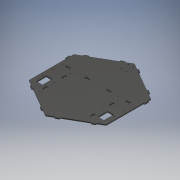
# Autodesk Inventor part: BA20
Saved by Autodesk Inventor 2017 (Build 210142000, 142)
## iProperties
Created: 2019-06-03
Part Number: BA20
Material: Polyethylene, High Density
Document SubType Name: Modeling
Designer: Dell
Density: 0.952 g/cm^3
Appearance: Smooth - Black
Mass: 1382.1 g
Surface Area: 4727.34 cm^2
Volume: 1451.78 cm^3
Author: Dell
Autodesk Inventor part; units mm, degrees
ref_plane "YZ Plane" through (0, 0, 0) normal (1, 0, 0) x (0, 1, 0)
ref_plane "XZ Plane" through (0, 0, 0) normal (0, 1, 0) x (-1, 0, 0)
ref_plane "XY Plane" through (0, 0, 0) normal (0, 0, 1) x (1, 0, 0)
sketch "Sketch1" plane through (0, 0, 0) normal (0, 0, 1) x (1, 0, 0)
  line L0 (0, 303.5592) -> (262.89, 151.7796) construction
  line L1 (262.89, 151.7796) -> (262.89, -151.7796) construction
  line L2 (262.89, -151.7796) -> (0, -303.5592) construction
  line L3 (0, -303.5592) -> (-262.89, -151.7796) construction
  line L4 (-262.89, -151.7796) -> (-262.89, 151.7796) construction
  line L5 (-262.89, 151.7796) -> (0, 303.5592) construction
  line L6 (0, 296.2269) -> (256.54, 148.1134)
  line L7 (256.54, 148.1134) -> (256.54, -148.1134)
  line L8 (256.54, -148.1134) -> (0, -296.2269)
  line L9 (0, -296.2269) -> (-256.54, -148.1134)
  line L10 (-256.54, -148.1134) -> (-256.54, 148.1134)
  line L11 (-256.54, 148.1134) -> (0, 296.2269)
  point P0 (0, 0)
  point P1 (0, 0)
  point P2 (262.89, 0)
  dimension "d0" = 525.78
  dimension "d1" = 6.35
  constraints: 24 end point, 1 coincident, 1 horizontal alignment, 1 midpoint, 18 other
  measures "d0" distance between parallel lines of L1 L4
  measures "d1" distance between parallel lines of L4 L10
extrude "Extrusion1" add sketch "Sketch1" along normal blind 6.35
sketch "Sketch2" plane through (0, 0, 6.35) normal (0, 0, 1) x (1, 0, 0)
  line L0 (-212.09, 56.5296) -> (-186.69, 56.5296)
  line L1 (-186.69, 56.5296) -> (-186.69, 50.1796)
  line L2 (-186.69, 50.1796) -> (-212.09, 50.1796)
  line L3 (-212.09, 50.1796) -> (-212.09, 56.5296)
  line L4 (256.54, 148.1134) -> (0, 296.2269) construction
  line L5 (0, 296.2269) -> (-256.54, 148.1134) construction
  line L6 (-256.54, 148.1134) -> (-256.54, -148.1134) construction
  line L7 (-256.54, -148.1134) -> (0, -296.2269) construction
  line L8 (0, -296.2269) -> (256.54, -148.1134) construction
  line L9 (256.54, -148.1134) -> (256.54, 148.1134) construction
  line L10 (-262.89, 151.7796) -> (0, 303.5592) construction
  line L11 (0, 303.5592) -> (262.89, 151.7796) construction
  line L12 (262.89, 151.7796) -> (262.89, -151.7796) construction
  line L13 (262.89, -151.7796) -> (0, -303.5592) construction
  line L14 (0, -303.5592) -> (-262.89, -151.7796) construction
  line L15 (-262.89, -151.7796) -> (-262.89, 151.7796) construction
  line L16 (-85.09, 50.1796) -> (-59.69, 50.1796)
  line L17 (-59.69, 50.1796) -> (-59.69, 56.5296)
  line L18 (-59.69, 56.5296) -> (-85.09, 56.5296)
  line L19 (-85.09, 56.5296) -> (-85.09, 50.1796)
  line L20 (0, 0) -> (0, 303.5592) construction
  line L21 (212.09, 56.5296) -> (186.69, 56.5296)
  line L22 (186.69, 56.5296) -> (186.69, 50.1796)
  line L23 (186.69, 50.1796) -> (212.09, 50.1796)
  line L24 (212.09, 50.1796) -> (212.09, 56.5296)
  line L25 (85.09, 50.1796) -> (59.69, 50.1796)
  line L26 (59.69, 50.1796) -> (59.69, 56.5296)
  line L27 (59.69, 56.5296) -> (85.09, 56.5296)
  line L28 (85.09, 56.5296) -> (85.09, 50.1796)
  point P0 (-186.69, 53.3546)
  point P1 (-85.09, 53.3546)
  point P2 (186.69, 53.3546)
  point P3 (85.09, 53.3546)
  dimension "d4" = 6.35
  dimension "d6" = 50.8
  dimension "d7" = 6.35
  dimension "d8" = 25.4
  dimension "d9" = 25.4
  dimension "d10" = 101.6
  dimension "d13" = 101.6
  constraints: 46 end point, 10 symmetric about line, 4 parallel, 2 horizontal, 2 horizontal alignment, 2 midpoint, 2 perpendicular, 1 vertical, 5 other
  measures "d4" distance between parallel lines of L5 L10
  measures "d6" distance between parallel lines of L15 L3
  measures "d7" distance of L2.end L0.start
  measures "d8" distance of L0.start L0.end
  measures "d9" distance of L17.end L18.end
  measures "d10" distance between parallel lines of L1 L19
  measures "d13" distance from line of L10.start L2
extrude "Extrusion2" cut sketch "Sketch2" against normal through all
sketch "Sketch3" plane through (0, 0, 6.35) normal (0, 0, 1) x (1, 0, 0)
  line L0 (-161.29, -0.6204) -> (-154.94, -0.6204)
  line L1 (-154.94, -0.6204) -> (-154.94, -26.0204)
  line L2 (-154.94, -26.0204) -> (-161.29, -26.0204)
  line L3 (-161.29, -26.0204) -> (-161.29, -0.6204)
  line L4 (-186.69, 50.1796) -> (-212.09, 50.1796) projected
  line L5 (-161.29, -127.6204) -> (-154.94, -127.6204)
  line L6 (-154.94, -127.6204) -> (-154.94, -153.0204)
  line L7 (-154.94, -153.0204) -> (-161.29, -153.0204)
  line L8 (-161.29, -153.0204) -> (-161.29, -127.6204)
  line L9 (-256.54, 148.1134) -> (-256.54, -148.1134) projected
  line L10 (0, 0) -> (0, 56.7776) construction
  line L11 (161.29, -0.6204) -> (154.94, -0.6204)
  line L12 (154.94, -0.6204) -> (154.94, -26.0204)
  line L13 (154.94, -26.0204) -> (161.29, -26.0204)
  line L14 (161.29, -26.0204) -> (161.29, -0.6204)
  line L15 (161.29, -127.6204) -> (154.94, -127.6204)
  line L16 (154.94, -127.6204) -> (154.94, -153.0204)
  line L17 (154.94, -153.0204) -> (161.29, -153.0204)
  line L18 (161.29, -153.0204) -> (161.29, -127.6204)
  dimension "d14" = 6.35
  dimension "d15" = 25.4
  dimension "d16" = 50.8
  dimension "d17" = 6.35
  dimension "d18" = 25.4
  dimension "d19" = 101.6
  dimension "d20" = 95.25
  constraints: 34 end point, 8 symmetric about line, 4 parallel, 2 horizontal, 2 perpendicular, 1 vertical, 1 vertical alignment
  measures "d14" distance of L1.end L2.end
  measures "d15" distance of L2.end L0.start
  measures "d16" distance between parallel lines of L0 L4
  measures "d17" distance of L6.end L7.end
  measures "d18" distance of L5.end L6.end
  measures "d19" distance of L5.start L2.end
  measures "d20" distance between parallel lines of L9 L3
extrude "Extrusion3" cut sketch "Sketch3" along normal through all both and the other way through all
sketch "Sketch4" plane through (0, 0, 6.35) normal (0, 0, 1) x (1, 0, 0)
  line L0 (-264.16, 126.3796) -> (-256.54, 126.3796)
  line L1 (-256.54, 126.3796) -> (-256.54, 100.9796)
  line L2 (-256.54, 100.9796) -> (-264.16, 100.9796)
  line L3 (-264.16, 100.9796) -> (-264.16, 126.3796)
  line L4 (-220.0682, -177.9693) -> (-216.2582, -171.3702)
  line L5 (-216.2582, -171.3702) -> (-194.2611, -184.0702)
  line L6 (-194.2611, -184.0702) -> (-198.0711, -190.6693)
  line L7 (-198.0711, -190.6693) -> (-220.0682, -177.9693)
  line L8 (-62.2789, -260.2702) -> (-66.0889, -266.8693)
  line L9 (-66.0889, -266.8693) -> (-44.0918, -279.5693)
  line L10 (-44.0918, -279.5693) -> (-40.2818, -272.9702)
  line L11 (-40.2818, -272.9702) -> (-62.2789, -260.2702)
  line L12 (-256.54, 148.1134) -> (-256.54, -148.1134) projected
  line L13 (-256.54, -148.1134) -> (0, -296.2269) projected
  line L14 (-196.1661, -187.3697) -> (-64.1839, -263.5697) construction
  line L15 (-130.175, -225.4697) -> (-128.27, -222.1702)
  line L16 (-212.09, 56.5296) -> (-186.69, 56.5296) projected
  line L17 (-186.69, 50.1796) -> (-212.09, 50.1796) projected
  line L18 (0, 0) -> (-92.269, 0) construction
  line L19 (-220.0682, 177.9693) -> (-216.2582, 171.3702)
  line L20 (-216.2582, 171.3702) -> (-194.2611, 184.0702)
  line L21 (-194.2611, 184.0702) -> (-198.0711, 190.6693)
  line L22 (-198.0711, 190.6693) -> (-220.0682, 177.9693)
  line L23 (-62.2789, 260.2702) -> (-66.0889, 266.8693)
  line L24 (-66.0889, 266.8693) -> (-44.0918, 279.5693)
  line L25 (-44.0918, 279.5693) -> (-40.2818, 272.9702)
  line L26 (-40.2818, 272.9702) -> (-62.2789, 260.2702)
  line L27 (-256.54, 148.1134) -> (0, 296.2269)
  line L28 (-196.1661, 187.3697) -> (-64.1839, 263.5697) construction
  line L29 (-130.175, 225.4697) -> (-128.27, 222.1702)
  line L30 (0, 0) -> (0, -66.9145) construction
  line L31 (264.16, 126.3796) -> (256.54, 126.3796)
  line L32 (256.54, 126.3796) -> (256.54, 100.9796)
  line L33 (256.54, 100.9796) -> (264.16, 100.9796)
  line L34 (264.16, 100.9796) -> (264.16, 126.3796)
  line L35 (220.0682, -177.9693) -> (216.2582, -171.3702)
  line L36 (216.2582, -171.3702) -> (194.2611, -184.0702)
  line L37 (194.2611, -184.0702) -> (198.0711, -190.6693)
  line L38 (198.0711, -190.6693) -> (220.0682, -177.9693)
  line L39 (62.2789, -260.2702) -> (66.0889, -266.8693)
  line L40 (66.0889, -266.8693) -> (44.0918, -279.5693)
  line L41 (44.0918, -279.5693) -> (40.2818, -272.9702)
  line L42 (40.2818, -272.9702) -> (62.2789, -260.2702)
  line L43 (256.54, 148.1134) -> (256.54, -148.1134)
  line L44 (196.1661, -187.3697) -> (64.1839, -263.5697) construction
  line L45 (130.175, -225.4697) -> (128.27, -222.1702)
  line L46 (212.09, 56.5296) -> (186.69, 56.5296)
  line L47 (186.69, 50.1796) -> (212.09, 50.1796)
  line L48 (198.0711, 190.6693) -> (220.0682, 177.9693)
  line L49 (220.0682, 177.9693) -> (216.2582, 171.3702)
  line L50 (216.2582, 171.3702) -> (194.2611, 184.0702)
  line L51 (194.2611, 184.0702) -> (198.0711, 190.6693)
  line L52 (130.175, 225.4697) -> (128.27, 222.1702)
  line L53 (196.1661, 187.3697) -> (64.1839, 263.5697) construction
  line L54 (62.2789, 260.2702) -> (66.0889, 266.8693)
  line L55 (40.2818, 272.9702) -> (62.2789, 260.2702)
  line L56 (66.0889, 266.8693) -> (44.0918, 279.5693)
  line L57 (44.0918, 279.5693) -> (40.2818, 272.9702)
  point P0 (92.269, 0)
  dimension "d23" = 7.62
  dimension "d24" = 25.4
  dimension "d25" = 7.62
  dimension "d26" = 25.4
  dimension "d27" = 25.4
  dimension "d28" = 7.62
  dimension "d29" = 152.4
  dimension "d31" = 50.8
  constraints: 108 end point, 48 symmetric about line, 10 point on line, 6 parallel, 4 midpoint, 4 perpendicular, 2 horizontal, 1 coincident, 1 vertical
  measures "d23" distance of L1.end L2.end
  measures "d24" distance of L0.end L1.end
  measures "d25" distance of L4.start L4.end
  measures "d26" distance of L4.end L5.end
  measures "d27" distance of L8.end L9.end
  measures "d28" distance of L8.start L8.end
  measures "d29" distance of L14.start L14.end
  measures "d31" distance from line of L2.end L17
extrude "Extrusion4" add sketch "Sketch4" against normal blind 6.35
sketch "Sketch5" plane through (0, 0, 6.35) normal (0, 0, 1) x (1, 0, 0)
  line L0 (-15.15, 270.8269) -> (15.15, 270.8269) construction
  line L1 (15.15, 270.8269) -> (15.15, 225.2269) construction
  line L2 (15.15, 225.2269) -> (-15.15, 225.2269) construction
  line L3 (-15.15, 225.2269) -> (-15.15, 270.8269) construction
  circle A0 centre (-15.15, 270.8269) radius 3
  circle A1 centre (15.15, 270.8269) radius 3
  circle A2 centre (15.15, 225.2269) radius 3
  circle A3 centre (-15.15, 225.2269) radius 3
  point P0 (0, 0)
  point P1 (0, 270.8269)
  point P2 (0, 296.2269)
  dimension "d34" = 45.6
  dimension "d35" = 30.3
  dimension "d36" = 25.4
  dimension "d37" = 6
  dimension "d38" = 6
  dimension "d39" = 6
  dimension "d40" = 6
  constraints: 8 end point, 4 centre point, 4 coincident, 2 parallel, 1 horizontal, 1 midpoint, 1 perpendicular, 1 vertical alignment
  measures "d34" distance of L0.end L1.end
  measures "d35" distance of L0.start L0.end
  measures "d36" distance from line of point (0, 296.227) L0
  measures "d37" diameter of A0
  measures "d38" diameter of A1
  measures "d39" diameter of A2
  measures "d40" diameter of A3
extrude "Extrusion5" cut sketch "Sketch5" against normal through all
sketch "Sketch6" plane through (0, 0, 6.35) normal (0, 0, 1) x (1, 0, 0)
  circle A0 centre (-207.1647, -181.0197) radius 2.25
  circle A1 centre (-260.35, 113.6796) radius 2.25
  circle A2 centre (-234.315, 53.3546) radius 2.25
  circle A3 centre (-135.89, 53.3546) radius 2.25
  circle A4 centre (0, 53.3546) radius 2.25
  circle A5 centre (-158.115, -178.9798) radius 2.25
  circle A6 centre (-158.115, -76.8204) radius 2.25
  circle A7 centre (-158.115, 26.3671) radius 2.25
  circle A8 centre (-53.1853, -269.9197) radius 2.25
  circle A9 centre (-207.1647, 181.0197) radius 2.25
  circle A10 centre (-53.1853, 269.9197) radius 2.25
  line L0 (-161.29, -0.6204) -> (-154.94, -0.6204) projected
  line L1 (-59.69, 56.5296) -> (-59.69, 50.1796) projected
  line L2 (-264.16, 126.3796) -> (-264.16, 100.9796) projected
  line L3 (-256.54, 126.3796) -> (-264.16, 126.3796) projected
  line L4 (-212.09, 50.1796) -> (-212.09, 56.5296) projected
  line L5 (-212.09, 53.3546) -> (-256.54, 53.3546)
  line L6 (-256.54, 100.9796) -> (-256.54, -148.1134) projected
  line L7 (-186.69, 56.5296) -> (-186.69, 50.1796) projected
  line L8 (-186.69, 53.3546) -> (-85.09, 53.3546)
  line L9 (-85.09, 50.1796) -> (-85.09, 56.5296) projected
  line L10 (-158.115, -0.6204) -> (-158.115, 53.3546)
  line L11 (-161.29, -26.0204) -> (-154.94, -26.0204) projected
  line L12 (-158.115, -26.0204) -> (-158.115, -127.6204)
  line L13 (-161.29, -127.6204) -> (-154.94, -127.6204) projected
  line L14 (-154.94, -153.0204) -> (-161.29, -153.0204) projected
  line L15 (-158.115, -153.0204) -> (-158.115, -204.9391)
  line L16 (-62.2789, -260.2702) -> (-194.2611, -184.0702) projected
  line L17 (-216.2582, -171.3702) -> (-220.0682, -177.9693) projected
  line L18 (-218.1632, -174.6697) -> (-207.1647, -181.0197) construction
  line L19 (-207.1647, -181.0197) -> (-209.0697, -184.3193) construction
  line L20 (-220.0682, -177.9693) -> (-198.0711, -190.6693) projected
  line L21 (-216.2582, 171.3702) -> (-220.0682, 177.9693) projected
  line L22 (-218.1632, 174.6697) -> (-207.1647, 181.0197) construction
  line L23 (-207.1647, 181.0197) -> (-209.0697, 184.3193) construction
  line L24 (-220.0682, 177.9693) -> (-198.0711, 190.6693) construction
  line L25 (-62.2789, 260.2702) -> (-66.0889, 266.8693) projected
  line L26 (-64.1839, 263.5697) -> (-53.1853, 269.9197) construction
  line L27 (-53.1853, 269.9197) -> (-55.0903, 273.2193) construction
  line L28 (-44.0918, 279.5693) -> (-66.0889, 266.8693) projected
  line L29 (-62.2789, -260.2702) -> (-66.0889, -266.8693) projected
  line L30 (-64.1839, -263.5697) -> (-53.1853, -269.9197) construction
  line L31 (-53.1853, -269.9197) -> (-55.0903, -273.2193) construction
  line L32 (-66.0889, -266.8693) -> (-44.0918, -279.5693) projected
  line L33 (0, 0) -> (0, -97.3082) construction
  circle A11 centre (207.1647, -181.0197) radius 2.25
  circle A12 centre (260.35, 113.6796) radius 2.25
  circle A13 centre (234.315, 53.3546) radius 2.25
  circle A14 centre (135.89, 53.3546) radius 2.25
  circle A15 centre (158.115, -178.9798) radius 2.25
  circle A16 centre (158.115, -76.8204) radius 2.25
  circle A17 centre (158.115, 26.3671) radius 2.25
  circle A18 centre (53.1853, -269.9197) radius 2.25
  circle A19 centre (207.1647, 181.0197) radius 2.25
  circle A20 centre (53.1853, 269.9197) radius 2.25
  line L34 (161.29, -0.6204) -> (154.94, -0.6204)
  line L35 (59.69, 56.5296) -> (59.69, 50.1796)
  line L36 (264.16, 126.3796) -> (264.16, 100.9796)
  line L37 (256.54, 126.3796) -> (264.16, 126.3796)
  line L38 (212.09, 50.1796) -> (212.09, 56.5296)
  line L39 (212.09, 53.3546) -> (256.54, 53.3546)
  line L40 (256.54, 100.9796) -> (256.54, -148.1134)
  line L41 (186.69, 56.5296) -> (186.69, 50.1796)
  line L42 (186.69, 53.3546) -> (85.09, 53.3546)
  line L43 (85.09, 50.1796) -> (85.09, 56.5296)
  line L44 (158.115, -0.6204) -> (158.115, 53.3546)
  line L45 (161.29, -26.0204) -> (154.94, -26.0204)
  line L46 (158.115, -26.0204) -> (158.115, -127.6204)
  line L47 (161.29, -127.6204) -> (154.94, -127.6204)
  line L48 (154.94, -153.0204) -> (161.29, -153.0204)
  line L49 (158.115, -153.0204) -> (158.115, -204.9391)
  line L50 (62.2789, -260.2702) -> (194.2611, -184.0702)
  line L51 (216.2582, -171.3702) -> (220.0682, -177.9693)
  line L52 (218.1632, -174.6697) -> (207.1647, -181.0197) construction
  line L53 (207.1647, -181.0197) -> (209.0697, -184.3193) construction
  line L54 (220.0682, -177.9693) -> (198.0711, -190.6693)
  line L55 (216.2582, 171.3702) -> (220.0682, 177.9693)
  line L56 (218.1632, 174.6697) -> (207.1647, 181.0197) construction
  line L57 (207.1647, 181.0197) -> (209.0697, 184.3193) construction
  line L58 (220.0682, 177.9693) -> (198.0711, 190.6693) construction
  line L59 (62.2789, 260.2702) -> (66.0889, 266.8693)
  line L60 (64.1839, 263.5697) -> (53.1853, 269.9197) construction
  line L61 (53.1853, 269.9197) -> (55.0903, 273.2193) construction
  line L62 (44.0918, 279.5693) -> (66.0889, 266.8693)
  line L63 (62.2789, -260.2702) -> (66.0889, -266.8693)
  line L64 (64.1839, -263.5697) -> (53.1853, -269.9197) construction
  line L65 (53.1853, -269.9197) -> (55.0903, -273.2193) construction
  line L66 (66.0889, -266.8693) -> (44.0918, -279.5693)
  point P0 (-59.69, 53.3546)
  point P1 (-264.16, 113.6796)
  point P2 (-260.35, 126.3796)
  point P3 (-135.89, 53.3546)
  point P4 (-234.315, 53.3546)
  point P5 (59.69, 53.3546)
  point P6 (264.16, 113.6796)
  point P7 (260.35, 126.3796)
  point P8 (158.115, -76.8204)
  point P9 (135.89, 53.3546)
  point P10 (234.315, 53.3546)
  dimension "d43" = 4.5
  dimension "d44" = 4.5
  dimension "d45" = 4.5
  dimension "d46" = 4.5
  dimension "d47" = 4.5
  dimension "d53" = 4.5
  dimension "d54" = 4.5
  dimension "d55" = 4.5
  dimension "d56" = 4.5
  dimension "d57" = 4.5
  dimension "d58" = 4.5
  constraints: 94 end point, 70 symmetric about line, 23 midpoint, 21 centre point, 10 coincident, 9 perpendicular, 8 point on line, 5 vertical alignment, 4 horizontal alignment, 1 horizontal, 1 vertical, 10 other
  measures "d43" diameter of A0
  measures "d44" diameter of A1
  measures "d45" diameter of A2
  measures "d46" diameter of A3
  measures "d47" diameter of A4
  measures "d53" diameter of A5
  measures "d54" diameter of A6
  measures "d55" diameter of A7
  measures "d56" diameter of A8
  measures "d57" diameter of A9
  measures "d58" diameter of A10
extrude "Extrusion6" cut sketch "Sketch6" against normal through all
sketch "Sketch7" plane through (0, 0, 6.35) normal (0, 0, 1) x (1, 0, 0)
  circle A0 centre (-238.84, -7.2826) radius 2.5
  circle A1 centre (-238.84, -74.7826) radius 2.5
  line L0 (-186.69, 50.1796) -> (-212.09, 50.1796) projected
  line L1 (-256.54, 100.9796) -> (-256.54, -148.1134) projected
  line L2 (0, 0) -> (0, 120.453)
  circle A2 centre (238.84, -7.2826) radius 2.5
  circle A3 centre (238.84, -74.7826) radius 2.5
  line L3 (186.69, 50.1796) -> (212.09, 50.1796)
  line L4 (256.54, 100.9796) -> (256.54, -148.1134)
  dimension "d61" = 5
  dimension "d62" = 5
  dimension "d63" = 57.4622
  dimension "d64" = 17.7
  dimension "d65" = 67.5
  constraints: 6 end point, 6 symmetric about line, 4 centre point, 1 vertical, 1 vertical alignment, 2 other
  measures "d61" diameter of A0
  measures "d62" diameter of A1
  measures "d63" distance from line of L0 A0.centre
  measures "d64" distance from line of L1 A0.centre
  measures "d65" distance of A1.centre A0.centre
extrude "Extrusion7" cut sketch "Sketch7" against normal through all
sketch "Sketch8" plane through (0, 0, 6.35) normal (0, 0, 1) x (1, 0, 0)
  circle A0 centre (238.84, -7.2826) radius 2.5 construction
  circle A1 centre (-238.84, -7.2826) radius 2.5 construction
  circle A2 centre (-238.84, -74.7826) radius 2.5 construction
  circle A3 centre (238.84, -74.7826) radius 2.5 construction
  circle A4 centre (207.1647, 181.0197) radius 2.25 construction
  circle A5 centre (207.1647, -181.0197) radius 2.25 construction
  circle A6 centre (158.115, -76.8204) radius 2.25 construction
  circle A7 centre (234.315, 53.3546) radius 2.25 construction
  circle A8 centre (158.115, 26.3671) radius 2.25 construction
  circle A9 centre (-207.1647, 181.0197) radius 2.25 construction
  circle A10 centre (-158.115, 26.3671) radius 2.25 construction
  circle A11 centre (-158.115, -178.9798) radius 2.25 construction
  circle A12 centre (-135.89, 53.3546) radius 2.25 construction
  circle A13 centre (-260.35, 113.6796) radius 2.25 construction
  circle A14 centre (-207.1647, -181.0197) radius 2.25 construction
  circle A15 centre (-234.315, 53.3546) radius 2.25 construction
  circle A16 centre (0, 53.3546) radius 2.25 construction
  circle A17 centre (-158.115, -76.8204) radius 2.25 construction
  circle A18 centre (-53.1853, -269.9197) radius 2.25 construction
  circle A19 centre (-53.1853, 269.9197) radius 2.25 construction
  circle A20 centre (135.89, 53.3546) radius 2.25 construction
  circle A21 centre (260.35, 113.6796) radius 2.25 construction
  circle A22 centre (53.1853, -269.9197) radius 2.25 construction
  circle A23 centre (158.115, -178.9798) radius 2.25 construction
  circle A24 centre (53.1853, 269.9197) radius 2.25 construction
  circle A25 centre (15.15, 225.2269) radius 3 construction
  circle A26 centre (-15.15, 270.8269) radius 3 construction
  circle A27 centre (15.15, 270.8269) radius 3 construction
  circle A28 centre (-15.15, 225.2269) radius 3 construction
  line L0 (161.29, -0.6204) -> (161.29, -26.0204) construction
  line L1 (161.29, -26.0204) -> (154.94, -26.0204) construction
  line L2 (154.94, -26.0204) -> (154.94, -0.6204) construction
  line L3 (154.94, -0.6204) -> (161.29, -0.6204) construction
  line L4 (-154.94, -0.6204) -> (-154.94, -26.0204) construction
  line L5 (-154.94, -26.0204) -> (-161.29, -26.0204) construction
  line L6 (-161.29, -26.0204) -> (-161.29, -0.6204) construction
  line L7 (-161.29, -0.6204) -> (-154.94, -0.6204) construction
  line L8 (-154.94, -127.6204) -> (-154.94, -153.0204) construction
  line L9 (-154.94, -153.0204) -> (-161.29, -153.0204) construction
  line L10 (-161.29, -153.0204) -> (-161.29, -127.6204) construction
  line L11 (-161.29, -127.6204) -> (-154.94, -127.6204) construction
  line L12 (161.29, -127.6204) -> (161.29, -153.0204) construction
  line L13 (161.29, -153.0204) -> (154.94, -153.0204) construction
  line L14 (154.94, -153.0204) -> (154.94, -127.6204) construction
  line L15 (154.94, -127.6204) -> (161.29, -127.6204) construction
  line L16 (85.09, 56.5296) -> (85.09, 50.1796) construction
  line L17 (85.09, 50.1796) -> (59.69, 50.1796) construction
  line L18 (59.69, 50.1796) -> (59.69, 56.5296) construction
  line L19 (59.69, 56.5296) -> (85.09, 56.5296) construction
  line L20 (-212.09, 50.1796) -> (-212.09, 56.5296) construction
  line L21 (-212.09, 56.5296) -> (-186.69, 56.5296) construction
  line L22 (-186.69, 56.5296) -> (-186.69, 50.1796) construction
  line L23 (-186.69, 50.1796) -> (-212.09, 50.1796) construction
  line L24 (-59.69, 56.5296) -> (-59.69, 50.1796) construction
  line L25 (-59.69, 50.1796) -> (-85.09, 50.1796) construction
  line L26 (-85.09, 50.1796) -> (-85.09, 56.5296) construction
  line L27 (-85.09, 56.5296) -> (-59.69, 56.5296) construction
  line L28 (212.09, 50.1796) -> (186.69, 50.1796) construction
  line L29 (186.69, 50.1796) -> (186.69, 56.5296) construction
  line L30 (186.69, 56.5296) -> (212.09, 56.5296) construction
  line L31 (212.09, 56.5296) -> (212.09, 50.1796) construction
  line L32 (256.54, 148.1134) -> (216.2582, 171.3702) construction
  line L33 (216.2582, 171.3702) -> (220.0682, 177.9693) construction
  line L34 (220.0682, 177.9693) -> (198.0711, 190.6693) construction
  line L35 (198.0711, 190.6693) -> (194.2611, 184.0702) construction
  line L36 (194.2611, 184.0702) -> (62.2789, 260.2702) construction
  line L37 (62.2789, 260.2702) -> (66.0889, 266.8693) construction
  line L38 (66.0889, 266.8693) -> (44.0918, 279.5693) construction
  line L39 (44.0918, 279.5693) -> (40.2818, 272.9702) construction
  line L40 (40.2818, 272.9702) -> (0, 296.2269) construction
  line L41 (0, 296.2269) -> (-40.2818, 272.9702) construction
  line L42 (-40.2818, 272.9702) -> (-44.0918, 279.5693) construction
  line L43 (-44.0918, 279.5693) -> (-66.0889, 266.8693) construction
  line L44 (-66.0889, 266.8693) -> (-62.2789, 260.2702) construction
  line L45 (-62.2789, 260.2702) -> (-194.2611, 184.0702) construction
  line L46 (-194.2611, 184.0702) -> (-198.0711, 190.6693) construction
  line L47 (-198.0711, 190.6693) -> (-220.0682, 177.9693) construction
  line L48 (-220.0682, 177.9693) -> (-216.2582, 171.3702) construction
  line L49 (-216.2582, 171.3702) -> (-256.54, 148.1134) construction
  line L50 (-256.54, 148.1134) -> (-256.54, 126.3796) construction
  line L51 (-256.54, 126.3796) -> (-264.16, 126.3796) construction
  line L52 (-264.16, 126.3796) -> (-264.16, 100.9796) construction
  line L53 (-264.16, 100.9796) -> (-256.54, 100.9796) construction
  line L54 (-256.54, 100.9796) -> (-256.54, -148.1134) construction
  line L55 (-256.54, -148.1134) -> (-216.2582, -171.3702) construction
  line L56 (-216.2582, -171.3702) -> (-220.0682, -177.9693) construction
  line L57 (-220.0682, -177.9693) -> (-198.0711, -190.6693) construction
  line L58 (-198.0711, -190.6693) -> (-194.2611, -184.0702) construction
  line L59 (-194.2611, -184.0702) -> (-62.2789, -260.2702) construction
  line L60 (-62.2789, -260.2702) -> (-66.0889, -266.8693) construction
  line L61 (-66.0889, -266.8693) -> (-44.0918, -279.5693) construction
  line L62 (-44.0918, -279.5693) -> (-40.2818, -272.9702) construction
  line L63 (-40.2818, -272.9702) -> (0, -296.2269) construction
  line L64 (0, -296.2269) -> (40.2818, -272.9702) construction
  line L65 (44.0918, -279.5693) -> (40.2818, -272.9702) construction
  line L66 (66.0889, -266.8693) -> (44.0918, -279.5693) construction
  line L67 (62.2789, -260.2702) -> (66.0889, -266.8693) construction
  line L68 (62.2789, -260.2702) -> (194.2611, -184.0702) construction
  line L69 (194.2611, -184.0702) -> (198.0711, -190.6693) construction
  line L70 (198.0711, -190.6693) -> (220.0682, -177.9693) construction
  line L71 (220.0682, -177.9693) -> (216.2582, -171.3702) construction
  line L72 (216.2582, -171.3702) -> (256.54, -148.1134) construction
  line L73 (256.54, -148.1134) -> (256.54, 100.9796) construction
  line L74 (264.16, 100.9796) -> (256.54, 100.9796) construction
  line L75 (264.16, 126.3796) -> (264.16, 100.9796) construction
  line L76 (256.54, 126.3796) -> (264.16, 126.3796) construction
  line L77 (256.54, 126.3796) -> (256.54, 148.1134) construction
  line L78 (-193.4394, 187.137) -> (-65.3457, 261.0919) construction
  line L79 (-65.3457, 261.0919) -> (-69.1557, 267.691) construction
  line L80 (-69.1557, 267.691) -> (-43.2701, 282.6361) construction
  line L81 (-43.2701, 282.6361) -> (-39.4601, 276.037) construction
  line L82 (-39.4601, 276.037) -> (0, 298.8193) construction
  line L83 (0, 298.8193) -> (39.4601, 276.037) construction
  line L84 (39.4601, 276.037) -> (43.2701, 282.6361) construction
  line L85 (43.2701, 282.6361) -> (69.1557, 267.691) construction
  line L86 (69.1557, 267.691) -> (65.3457, 261.0919) construction
  line L87 (65.3457, 261.0919) -> (193.4394, 187.137) construction
  line L88 (193.4394, 187.137) -> (197.2494, 193.7361) construction
  line L89 (197.2494, 193.7361) -> (223.135, 178.791) construction
  line L90 (223.135, 178.791) -> (219.325, 172.1919) construction
  line L91 (219.325, 172.1919) -> (258.7851, 149.4096) construction
  line L92 (258.7851, 149.4096) -> (258.7851, 128.6247) construction
  line L93 (258.7851, 128.6247) -> (266.4051, 128.6247) construction
  line L94 (266.4051, 128.6247) -> (266.4051, 98.7345) construction
  line L95 (266.4051, 98.7345) -> (258.7851, 98.7345) construction
  line L96 (258.7851, 98.7345) -> (258.7851, -149.4096) construction
  line L97 (258.7851, -149.4096) -> (219.325, -172.1919) construction
  line L98 (219.325, -172.1919) -> (223.135, -178.791) construction
  line L99 (223.135, -178.791) -> (197.2494, -193.7361) construction
  line L100 (197.2494, -193.7361) -> (193.4394, -187.137) construction
  line L101 (193.4394, -187.137) -> (65.3457, -261.0919) construction
  line L102 (65.3457, -261.0919) -> (69.1557, -267.691) construction
  line L103 (69.1557, -267.691) -> (43.2701, -282.6361) construction
  line L104 (43.2701, -282.6361) -> (39.4601, -276.037) construction
  line L105 (39.4601, -276.037) -> (0, -298.8193) construction
  line L106 (0, -298.8193) -> (-39.4601, -276.037) construction
  line L107 (-39.4601, -276.037) -> (-43.2701, -282.6361) construction
  line L108 (-43.2701, -282.6361) -> (-69.1557, -267.691) construction
  line L109 (-69.1557, -267.691) -> (-65.3457, -261.0919) construction
  line L110 (-65.3457, -261.0919) -> (-193.4394, -187.137) construction
  line L111 (-193.4394, -187.137) -> (-197.2494, -193.7361) construction
  line L112 (-197.2494, -193.7361) -> (-223.135, -178.791) construction
  line L113 (-223.135, -178.791) -> (-219.325, -172.1919) construction
  line L114 (-219.325, -172.1919) -> (-258.7851, -149.4096) construction
  line L115 (-258.7851, -149.4096) -> (-258.7851, 98.7345) construction
  line L116 (-258.7851, 98.7345) -> (-266.4051, 98.7345) construction
  line L117 (-266.4051, 98.7345) -> (-266.4051, 128.6247) construction
  line L118 (-266.4051, 128.6247) -> (-258.7851, 128.6247) construction
  line L119 (-258.7851, 128.6247) -> (-258.7851, 149.4096) construction
  line L120 (-258.7851, 149.4096) -> (-219.325, 172.1919) construction
  line L121 (-219.325, 172.1919) -> (-223.135, 178.791) construction
  line L122 (-223.135, 178.791) -> (-197.2494, 193.7361) construction
  line L123 (-197.2494, 193.7361) -> (-193.4394, 187.137) construction
  line L124 (-220.0682, -177.9693) -> (-216.2582, -171.3702) projected
  circle A29 centre (-219.325, -172.1919) radius 3.175
  line L125 (-62.2789, -260.2702) -> (-194.2611, -184.0702) projected
  circle A30 centre (-193.4394, -187.137) radius 3.175
  circle A31 centre (-258.7851, 98.7345) radius 3.175
  circle A32 centre (-258.7851, 128.6247) radius 3.175
  circle A33 centre (-219.325, 172.1919) radius 3.175
  circle A34 centre (-193.4394, 187.137) radius 3.175
  circle A35 centre (-65.3457, 261.0919) radius 3.175
  line L126 (0, 296.2269) -> (-40.2818, 272.9702) projected
  circle A36 centre (-39.4601, 276.037) radius 3.175
  circle A37 centre (39.4601, 276.037) radius 3.175
  circle A38 centre (65.3457, 261.0919) radius 3.175
  line L127 (62.2789, 260.2702) -> (194.2611, 184.0702) projected
  circle A39 centre (193.4394, 187.137) radius 3.175
  circle A40 centre (219.325, 172.1919) radius 3.175
  line L128 (256.54, 126.3796) -> (264.16, 126.3796) projected
  circle A41 centre (258.7851, 128.6247) radius 3.175
  circle A42 centre (258.7851, 98.7345) radius 3.175
  circle A43 centre (219.325, -172.1919) radius 3.175
  line L129 (194.2611, -184.0702) -> (198.0711, -190.6693) projected
  circle A44 centre (193.4394, -187.137) radius 3.175
  circle A45 centre (-65.3457, -261.0919) radius 3.175
  line L130 (-44.0918, -279.5693) -> (-40.2818, -272.9702) projected
  circle A46 centre (-39.4601, -276.037) radius 3.175
  circle A47 centre (39.4601, -276.037) radius 3.175
  line L131 (194.2611, -184.0702) -> (62.2789, -260.2702) projected
  circle A48 centre (65.3457, -261.0919) radius 3.175
  line L132 (-213.36, 57.7996) -> (-185.42, 57.7996)
  line L133 (-185.42, 57.7996) -> (-185.42, 48.9096)
  line L134 (-185.42, 48.9096) -> (-213.36, 48.9096)
  line L135 (-213.36, 48.9096) -> (-213.36, 57.7996)
  line L136 (-86.36, 57.7996) -> (-58.42, 57.7996)
  line L137 (-58.42, 57.7996) -> (-58.42, 48.9096)
  line L138 (-58.42, 48.9096) -> (-86.36, 48.9096)
  line L139 (-86.36, 48.9096) -> (-86.36, 57.7996)
  line L140 (58.42, 57.7996) -> (86.36, 57.7996)
  line L141 (86.36, 57.7996) -> (86.36, 48.9096)
  line L142 (86.36, 48.9096) -> (58.42, 48.9096)
  line L143 (58.42, 48.9096) -> (58.42, 57.7996)
  line L144 (185.42, 57.7996) -> (213.36, 57.7996)
  line L145 (213.36, 57.7996) -> (213.36, 48.9096)
  line L146 (213.36, 48.9096) -> (185.42, 48.9096)
  line L147 (185.42, 48.9096) -> (185.42, 57.7996)
  line L148 (153.67, 0.6496) -> (162.56, 0.6496)
  line L149 (162.56, 0.6496) -> (162.56, -27.2904)
  line L150 (162.56, -27.2904) -> (153.67, -27.2904)
  line L151 (153.67, -27.2904) -> (153.67, 0.6496)
  line L152 (153.67, -126.3504) -> (162.56, -126.3504)
  line L153 (162.56, -126.3504) -> (162.56, -154.2904)
  line L154 (162.56, -154.2904) -> (153.67, -154.2904)
  line L155 (153.67, -154.2904) -> (153.67, -126.3504)
  line L156 (-162.56, 0.6496) -> (-153.67, 0.6496)
  line L157 (-153.67, 0.6496) -> (-153.67, -27.2904)
  line L158 (-153.67, -27.2904) -> (-162.56, -27.2904)
  line L159 (-162.56, -27.2904) -> (-162.56, 0.6496)
  line L160 (-162.56, -126.3504) -> (-153.67, -126.3504)
  line L161 (-153.67, -126.3504) -> (-153.67, -154.2904)
  line L162 (-153.67, -154.2904) -> (-162.56, -154.2904)
  line L163 (-162.56, -154.2904) -> (-162.56, -126.3504)
  line L164 (-160.3149, -152.0453) -> (-155.9151, -152.0453)
  line L165 (-155.9151, -152.0453) -> (-155.9151, -128.5955)
  line L166 (-155.9151, -128.5955) -> (-160.3149, -128.5955)
  line L167 (-160.3149, -128.5955) -> (-160.3149, -152.0453)
  line L168 (-160.3149, -25.0453) -> (-155.9151, -25.0453)
  line L169 (-155.9151, -25.0453) -> (-155.9151, -1.5955)
  line L170 (-155.9151, -1.5955) -> (-160.3149, -1.5955)
  line L171 (-160.3149, -1.5955) -> (-160.3149, -25.0453)
  line L172 (-211.1149, 51.1547) -> (-187.6651, 51.1547)
  line L173 (-187.6651, 51.1547) -> (-187.6651, 55.5545)
  line L174 (-187.6651, 55.5545) -> (-211.1149, 55.5545)
  line L175 (-211.1149, 55.5545) -> (-211.1149, 51.1547)
  line L176 (-84.1149, 51.1547) -> (-60.6651, 51.1547)
  line L177 (-60.6651, 51.1547) -> (-60.6651, 55.5545)
  line L178 (-60.6651, 55.5545) -> (-84.1149, 55.5545)
  line L179 (-84.1149, 55.5545) -> (-84.1149, 51.1547)
  line L180 (60.6651, 51.1547) -> (84.1149, 51.1547)
  line L181 (84.1149, 51.1547) -> (84.1149, 55.5545)
  line L182 (84.1149, 55.5545) -> (60.6651, 55.5545)
  line L183 (60.6651, 55.5545) -> (60.6651, 51.1547)
  line L184 (187.6651, 51.1547) -> (211.1149, 51.1547)
  line L185 (211.1149, 51.1547) -> (211.1149, 55.5545)
  line L186 (211.1149, 55.5545) -> (187.6651, 55.5545)
  line L187 (187.6651, 55.5545) -> (187.6651, 51.1547)
  line L188 (160.3149, -25.0453) -> (160.3149, -1.5955)
  line L189 (160.3149, -1.5955) -> (155.9151, -1.5955)
  line L190 (155.9151, -1.5955) -> (155.9151, -25.0453)
  line L191 (155.9151, -25.0453) -> (160.3149, -25.0453)
  line L192 (160.3149, -152.0453) -> (160.3149, -128.5955)
  line L193 (160.3149, -128.5955) -> (155.9151, -128.5955)
  line L194 (155.9151, -128.5955) -> (155.9151, -152.0453)
  line L195 (155.9151, -152.0453) -> (160.3149, -152.0453)
  circle A49 centre (-160.3149, -152.0453) radius 3.175
  circle A50 centre (-155.9151, -152.0453) radius 3.175
  circle A51 centre (-155.9151, -128.5955) radius 3.175
  circle A52 centre (-160.3149, -128.5955) radius 3.175
  circle A53 centre (-160.3149, -25.0453) radius 3.175
  circle A54 centre (-160.3149, -1.5955) radius 3.175
  circle A55 centre (-155.9151, -25.0453) radius 3.175
  circle A56 centre (-155.9151, -1.5955) radius 3.175
  circle A57 centre (-211.1149, 51.1547) radius 3.175
  circle A58 centre (-211.1149, 55.5545) radius 3.175
  circle A59 centre (-187.6651, 51.1547) radius 3.175
  circle A60 centre (-187.6651, 55.5545) radius 3.175
  circle A61 centre (-84.1149, 55.5545) radius 3.175
  circle A62 centre (-84.1149, 51.1547) radius 3.175
  circle A63 centre (-60.6651, 55.5545) radius 3.175
  circle A64 centre (-60.6651, 51.1547) radius 3.175
  circle A65 centre (60.6651, 55.5545) radius 3.175
  circle A66 centre (60.6651, 51.1547) radius 3.175
  circle A67 centre (84.1149, 55.5545) radius 3.175
  circle A68 centre (84.1149, 51.1547) radius 3.175
  circle A69 centre (187.6651, 55.5545) radius 3.175
  circle A70 centre (187.6651, 51.1547) radius 3.175
  circle A71 centre (211.1149, 51.1547) radius 3.175
  circle A72 centre (211.1149, 55.5545) radius 3.175
  circle A73 centre (155.9151, -1.5955) radius 3.175
  circle A74 centre (160.3149, -1.5955) radius 3.175
  circle A75 centre (155.9151, -25.0453) radius 3.175
  circle A76 centre (160.3149, -25.0453) radius 3.175
  circle A77 centre (155.9151, -152.0453) radius 3.175
  circle A78 centre (155.9151, -128.5955) radius 3.175
  circle A79 centre (160.3149, -128.5955) radius 3.175
  circle A80 centre (160.3149, -152.0453) radius 3.175
  point P0 (0, 0)
  point P1 (-158.115, -0.6204)
  point P2 (-158.115, 0.6496)
  point P3 (-158.115, -127.6204)
  point P4 (-158.115, -126.3504)
  point P5 (158.115, -127.6204)
  point P6 (158.115, -126.3504)
  point P7 (158.115, -0.6204)
  point P8 (158.115, 0.6496)
  point P9 (72.39, 56.5296)
  point P10 (72.39, 57.7996)
  point P11 (199.39, 56.5296)
  point P12 (199.39, 57.7996)
  point P13 (-72.39, 56.5296)
  point P14 (-72.39, 57.7996)
  point P15 (-199.39, 56.5296)
  point P16 (-199.39, 57.7996)
  point P17 (-212.09, 53.3546)
  point P18 (-213.36, 53.3546)
  point P19 (-86.36, 53.3546)
  point P20 (-85.09, 53.3546)
  point P21 (59.69, 53.3546)
  point P22 (58.42, 53.3546)
  point P23 (185.42, 53.3546)
  point P24 (186.69, 53.3546)
  point P25 (153.67, -13.3204)
  point P26 (154.94, -13.3204)
  point P27 (-161.29, -13.3204)
  point P28 (-162.56, -13.3204)
  point P29 (-161.29, -140.3204)
  point P30 (-162.56, -140.3204)
  point P31 (154.94, -140.3204)
  point P32 (153.67, -140.3204)
  dimension "d68" = 6.35
  dimension "d78" = 6.35
  dimension "d79" = 6.35
  dimension "d80" = 6.35
  dimension "d81" = 6.35
  dimension "d82" = 6.35
  dimension "d83" = 6.35
  dimension "d84" = 6.35
  dimension "d85" = 6.35
  dimension "d69" = 8.89
  dimension "d70" = 27.94
  dimension "d71" = 27.94
  dimension "d72" = 27.94
  dimension "d73" = 27.94
  dimension "d74" = 27.94
  dimension "d75" = 27.94
  dimension "d76" = 8.89
  dimension "d77" = 8.89
  constraints: 220 end point, 52 coincident, 32 midpoint, 32 parallel, 16 perpendicular, 12 horizontal alignment, 9 vertical alignment, 8 horizontal, 3 point on line, 225 other
  measures "d69" distance between parallel lines of L134 L132
  measures "d70" distance between parallel lines of L133 L135
  measures "d71" distance of L136.start L136.end
  measures "d72" distance of L140.start L140.end
  measures "d73" distance of L144.start L144.end
  measures "d74" distance of L156.end L157.end
  measures "d75" distance of L160.end L161.end
  measures "d76" distance between parallel lines of L157 L159
  measures "d77" distance between parallel lines of L149 L151
extrude "Extrusion8" cut sketch "Sketch8" along normal through all both and the other way through all
sketch "Sketch9" plane through (0, 0, 6.35) normal (0, 0, 1) x (1, 0, 0)
  line L0 (-224.79, -67.2826) -> (-184.79, -67.2826)
  line L1 (-184.79, -67.2826) -> (-184.79, -132.2826)
  line L2 (-184.79, -132.2826) -> (-224.79, -132.2826)
  line L3 (-224.79, -132.2826) -> (-224.79, -67.2826)
  line L4 (-256.54, 96.4895) -> (-256.54, -148.1134) projected
  line L5 (0, 0) -> (0, -75.5419)
  line L6 (224.79, -67.2826) -> (184.79, -67.2826)
  line L7 (184.79, -67.2826) -> (184.79, -132.2826)
  line L8 (184.79, -132.2826) -> (224.79, -132.2826)
  line L9 (224.79, -132.2826) -> (224.79, -67.2826)
  line L10 (-224.79, 5.2174) -> (-224.79, -166.4443) construction
  line L11 (-256.54, -148.1134) -> (-220.1467, -169.1251) projected
  line L12 (-184.79, -99.7826) -> (-178.5985, -99.7826)
  point P0 (-256.54, 148.1134)
  dimension "d88" = 40
  dimension "d89" = 65
  dimension "d90" = 31.75
  dimension "d93" = 142.896
  dimension "d97" = 105
  constraints: 22 end point, 4 symmetric about line, 2 horizontal, 2 parallel, 2 point on line, 2 vertical, 1 midpoint, 1 perpendicular
  measures "d88" distance of L1.end L2.end
  measures "d89" distance of L0.end L1.end
  measures "d90" distance between parallel lines of L3 L4
  measures "d93" vertical distance of point (-256.54, 148.113) L10.start
  measures "d97" distance from line of L12 L10.start
extrude "Extrusion9" cut sketch "Sketch9" against normal through all
equation "\"d1\" = Panel_Thickness"
equation "\"d2\" = Panel_Thickness"
equation "\"d4\" = Panel_Thickness"
equation "\"d7\" = Panel_Thickness"
equation "\"d11\" = Panel_Thickness"
equation "\"d14\" = Panel_Thickness"
equation "\"d17\" = Panel_Thickness"
equation "\"d23\" = Panel_Thickness + Fit_Tolerance"
equation "\"d25\" = Panel_Thickness + Fit_Tolerance"
equation "\"d28\" = Panel_Thickness + Fit_Tolerance"
equation "\"d32\" = Panel_Thickness"
equation "\"d68\" = Tool_Dia"
equation "\"d78\" = Tool_Dia"
equation "\"d79\" = Tool_Dia"
equation "\"d80\" = Tool_Dia"
equation "\"d81\" = Tool_Dia"
equation "\"d82\" = Tool_Dia"
equation "\"d83\" = Tool_Dia"
equation "\"d84\" = Tool_Dia"
equation "\"d85\" = Tool_Dia"
equation "\"d69\" = Panel_Thickness + 2 * Fit_Tolerance"
equation "\"d76\" = Panel_Thickness + 2 * Fit_Tolerance"
equation "\"d77\" = Panel_Thickness + 2 * Fit_Tolerance"
equation "\"Panel_Thickness\" = 6.35"
equation "\"Fit_Tolerance\" = 1.27"
equation "\"Tool_Dia\" = 6.35"
body "Solid1"
